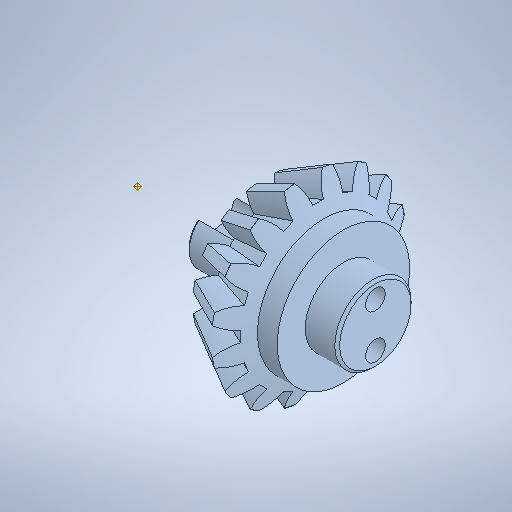
# Autodesk Inventor part: engrenage_secondaire
Saved by Autodesk Inventor 2025.1 (Build 291241000, 241)
## iProperties
Created: 2011-06-16
Part Number: engrenage_secondaire
Document SubType Name: Modeling
Designer: nguyenducthang
Density: 1 g/cm^3
Mass: 16.4156 g
Surface Area: 74.0163 cm^2
Volume: 16.4156 cm^3
Material: Generic
Appearance: Light Steel Blue
Author: nguyenducthang
Autodesk Inventor part; units mm, degrees
sketch "Sketch1" plane through (0, 0, 0) normal (0, 0, 1) x (1, 0, 0)
  line L0 (0, 0) -> (47.154021, 23.576958) construction
  circle A0 centre (0, 0) radius 40 construction
  line L1 (38, 13.442709) -> (34.882678, 19.677367)
  line L2 (56.339231, 30.40562) -> (13.1942, 8.833152) construction
  line L3 (26.161168, 14.759705) -> (34.837929, 19.654992)
  line L4 (28.330519, 11.481948) -> (46.75761, 20.695472) construction
  line L5 (29, 9.08203) -> (26.161168, 14.759705)
  line L6 (29, 9.08203) -> (29, 0)
  line L7 (34.882678, 19.677367) -> (34.837929, 19.654992)
  line L8 (35.777104, 17.888512) -> (35.777104, 0) construction
  line L9 (38, 13.442709) -> (38, 0)
  line L10 (0, 0) -> (29, 0) construction
  line L11 (40, 0) -> (43.641618, 0) construction
  line L12 (29, 0) -> (38, 0)
  dimension "d0" = 80
  dimension "d2" = 2
  dimension "d3" = 2.4
  dimension "d5" = 10
  dimension "d9" = 40
  dimension "d43" = 17.88851
  dimension "d47" = 35.7771
  dimension "d48" = 38
  dimension "d49" = 9
  dimension "d82" = 2.2229
  constraints: 26 end point, 5 perpendicular, 3 point on circle, 2 collinear, 2 horizontal, 2 parallel, 2 point on line, 1 centre point, 1 coincident, 1 tangent, 1 other
  measures "d0" diameter of A0
  measures "d2" distance between parallel lines of L2 L0
  measures "d3" distance between parallel lines of L4 L0
  measures "d5" distance between parallel lines of L5 L1
  measures "d9" distance from line of L1 A0.centre
  measures "d43" distance of L8.start L8.end
  measures "d47" distance from line of L8 A0.centre
  measures "d48" distance from line of L9 A0.centre
  measures "d49" distance between parallel lines of L6 L9
  measures "d82" distance between parallel lines of L8 L9
sketch "Sketch1 outline for Revolution1" plane through (0, 0, 0) normal (0, 0, 1) x (1, 0, 0)
  line L0 (34.882678, 19.677367) -> (38, 13.442709)
  line L1 (38, 13.442709) -> (38, 0)
  line L2 (38, 0) -> (29, 0)
  line L3 (29, 0) -> (29, 9.08203)
  line L4 (29, 9.08203) -> (26.161168, 14.759705)
  line L5 (26.161168, 14.759705) -> (34.837929, 19.654992)
  line L6 (34.837929, 19.654992) -> (34.882678, 19.677367)
revolve "Revolution1" add sketch "Sketch1 outline for Revolution1" angle 360 about axis through (29, 0, 0) along (1, 0, 0)
ref_plane "Work Plane2" through (36.660655, 15.999886, 0) normal (0.9165164, 0.3999971, 0) x (0, 0, 1)
ref_plane "Work Plane1" through (0, 0, 0) normal (0.9165164, 0.3999971, 0) x (0, 0, 1)
ref_plane "Work Plane5" through (35.777104, 17.888512, 0) normal (0.8944276, 0.4472128, 0) x (0, 0, 1)
ref_plane "Work Plane4" through (0, 0, 0) normal (0.8944276, 0.4472128, 0) x (0, 0, 1)
sketch "Sketch8" plane through (35.777104, 17.888512, 0) normal (0.8944276, 0.4472128, 0) x (0, 0, 1)
  ellipse E0 centre (0, 15.59998) end of major axis (19.677367, 15.59998) minor radius 17.59998
  line L0 (0, 15.59998) -> (0, -2)
  line L1 (0, -2) -> (-13.263403, -2) construction
  line L2 (3.441315, 0) -> (-9.391923, 0) construction
  line L3 (-1.756, -5.19782) -> (-1.756, 0) construction
  line L4 (-1.082471, 3.746493) -> (-1.082471, 1.872584) construction
  line L5 (-3.293908, -2.4) -> (-3.293908, -4.130276) construction
  line L6 (1.082471, 2.4) -> (-1.082471, 2.4)
  arc A0 (-3.293908, -2.4) -> (-1.082471, 2.4) centre (-10.050276, 3.622188) ccw
  arc A1 (1.082471, 2.4) -> (3.293908, -2.4) centre (10.050276, 3.622188) ccw
  line L7 (-3.293908, -2.4) -> (3.293908, -2.4)
  point P0 (-3.293908, -3.675872)
  dimension "d53" = 2
  dimension "d54" = 1.756
  dimension "d63" = 3.29391
  constraints: 16 end point, 5 point on circle, 3 parallel, 3 point on line, 3 symmetric about line, 2 centre point, 2 perpendicular, 1 horizontal, 1 vertical, 1 vertical alignment, 2 other
  measures "d53" distance between parallel lines of L1 L2
  measures "d54" distance between parallel lines of L3 L0
  measures "d63" distance between parallel lines of L0 L5
sketch "Sketch8 outline for Extrusion6" plane through (35.777104, 17.888512, 0) normal (0.8944276, 0.4472128, 0) x (0, 0, 1)
  arc A0 (-3.293908, -2.4) -> (-1.082471, 2.4) centre (-10.050276, 3.622188) ccw
  line L0 (-1.082471, 2.4) -> (1.082471, 2.4)
  arc A1 (1.082471, 2.4) -> (3.293908, -2.4) centre (10.050276, 3.622188) ccw
  line L1 (3.293908, -2.4) -> (-3.293908, -2.4)
extrude "Extrusion6" cut sketch "Sketch8 outline for Extrusion6" against normal blind 12 draft -2.86
pattern_circular "Circular Pattern2" count 16 over 360 about axis through (36.441339, 0, 0) along (1, 0, 0) of "Extrusion6"
ref_plane "Work Plane7" through (75, 0, 0) normal (1, 0, 0) x (0, 0, -1)
ref_plane "Work Plane6" through (35.777, 0, 0) normal (1, 0, 0) x (0, 0, -1)
sketch "Sketch11" plane through (35.777, 0, 0) normal (1, 0, 0) x (0, 0, -1)
  circle A0 centre (0, 0) radius 13.442709
  circle A1 centre (0, 0) radius 17.889
  dimension "d84" = 35.778
  constraints: 1 centre point, 1 coincident
  measures "d84" diameter of A1
sketch "Sketch12" plane through (0, 0, 0) normal (0, 0, 1) x (1, 0, 0)
  line L0 (38, -13.442709) -> (38, 13.442709)
  line L1 (29, -9.08203) -> (29, 9.08203)
  line L2 (38, 0) -> (38, 13.442709)
  line L3 (42, 13.442709) -> (42, 7.75)
  line L4 (42, 7.75) -> (48.5, 7.75)
  line L5 (48.5, 7.75) -> (48.5, 0)
  line L6 (48.5, 0) -> (38, 0)
  line L7 (29, 0) -> (26, 0)
  line L8 (26, 0) -> (26, 8)
  line L9 (26, 8) -> (29, 8)
  line L10 (29, 8) -> (29, 0)
  line L11 (38, 13.442709) -> (42, 13.442709)
  point P0 (0, 0)
  dimension "d89" = 6.5
  dimension "d90" = 8
  dimension "d91" = 3
  dimension "d96" = 7.75
  dimension "d130" = 4
  dimension "d131" = 13.44271
  constraints: 20 end point, 5 perpendicular, 2 midpoint, 2 parallel, 1 horizontal, 1 point on line, 1 vertical
  measures "d89" distance of L3.end L4.end
  measures "d90" distance of L7.end L8.end
  measures "d91" distance of L8.end L9.end
  measures "d96" distance between parallel lines of L6 L4
  measures "d130" distance between parallel lines of L3 L2
  measures "d131" distance between parallel lines of L6 L11
sketch "Sketch12 outline for Revolution3" plane through (0, 0, 0) normal (0, 0, 1) x (1, 0, 0)
  line L0 (26, 8) -> (26, 0)
  line L1 (29, 8) -> (26, 8)
  line L2 (29, 0) -> (29, 8)
  line L3 (26, 0) -> (29, 0)
  line L4 (48.5, 0) -> (48.5, 7.75)
  line L5 (38, 0) -> (48.5, 0)
  line L6 (38, 13.442709) -> (38, 0)
  line L7 (42, 13.442709) -> (38, 13.442709)
  line L8 (42, 7.75) -> (42, 13.442709)
  line L9 (48.5, 7.75) -> (42, 7.75)
revolve "Revolution3" add sketch "Sketch12 outline for Revolution3" angle 360 about axis through (48.5, 0, 0) along (-1, 0, 0)
sketch "Sketch13" plane through (26, 0, 0) normal (-1, 0, 0) x (0, 0, 1)
  circle A0 centre (0, 0) radius 5.8
  point P0 (0, 0)
  dimension "d93" = 11.6
  constraints: 1 centre point, 1 coincident
  measures "d93" diameter of A0
sketch "Sketch13 outline for Extrusion8" plane through (26, 0, 0) normal (-1, 0, 0) x (0, 0, 1)
  circle A0 centre (0, 0) radius 5.8
extrude "Extrusion8" add sketch "Sketch13 outline for Extrusion8" along normal blind 10
chamfer "Chamfer3" distance 0.5 angle 45 2 edges at (48.5, -7.75, 0) (16, 0, -5.8)
sketch "Esquisse20" plane through (48.5, 0, 0) normal (1, 0, 0) x (0, 0, -1)
  circle A0 centre (0, -4.5) radius 1.5
  circle A1 centre (0, 0) radius 13.442709
  line L0 (-13.442709, 0) -> (13.442709, 0)
  line L1 (0, 13.410383) -> (0, -13.410383)
  circle A2 centre (0, 4.5) radius 1.5
  dimension "d139" = 3
  dimension "d142" = 4.5
  constraints: 5 midpoint, 4 end point, 2 centre point, 2 point on circle, 1 coincident, 1 point on line, 1 symmetric about line, 1 vertical, 1 other
  measures "d139" diameter of A0
  measures "d142" distance of A1.centre point (0, -4.5)
hole "Perçage1" at (48.5, -4.5, 0) at (48.5, 4.5, 0) direction (-1, 0, 0) diameter 4 end through all
sketch "Esquisse22" plane through (16, 0, 0) normal (-1, 0, 0) x (0, 0, 1)
  arc A0 (1.953959, -4.926667) -> (-1.953959, -4.926667) centre (0, -4.5) ccw
  circle A1 centre (0, -4.5) radius 3.85
  circle A2 centre (0, 4.5) radius 2
  circle A3 centre (0, 4.5) radius 3.85
  point P0 (0, 0)
  dimension "d143" = 7.7
  constraints: 2 centre point, 2 coincident, 1 equal radius
  measures "d143" diameter of A1
sketch "Esquisse22 outline for Extrusion14" plane through (16, 0, 0) normal (-1, 0, 0) x (0, 0, 1)
  circle A0 centre (0, 4.5) radius 3.85
  circle A1 centre (0, -4.5) radius 3.85
extrude "Extrusion14" cut sketch "Esquisse22 outline for Extrusion14" against normal blind 15
body "Solid1"
